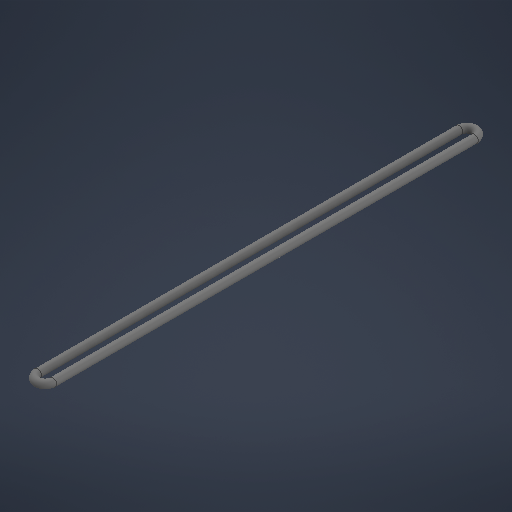
# Autodesk Inventor part: жгут сосало
Saved by Autodesk Inventor 2026.2 (Build 302298000, 298)
## iProperties
Created: 2026-01-20
Part Number: жгут сосало
Material: Типовые
Document SubType Name: Modeling
Designer: GameHD
Density: 1 g/cm^3
Appearance: По умолчанию
Author: GameHD
Autodesk Inventor part; units mm, degrees
ref_plane "YZ Plane" through (0, 0, 0) normal (1, 0, 0) x (0, 1, 0)
ref_plane "XZ Plane" through (0, 0, 0) normal (0, 1, 0) x (-1, 0, 0)
ref_plane "XY Plane" through (0, 0, 0) normal (0, 0, 1) x (1, 0, 0)
sketch "Эскиз1" plane through (0, 0, 0) normal (0, 0, 1) x (1, 0, 0)
  circle A0 centre (0, 0) radius 2.5
  dimension "d0" = 5
  constraints: 1 centre point, 1 coincident
  measures "d0" diameter of A0
sketch "Эскиз2" plane through (0, 0, 0) normal (0, 1, 0) x (-1, 0, 0)
  line L0 (0, 0) -> (-10, 0)
  line L1 (-5, 0) -> (-5, -275)
  line L2 (-5, 0) -> (270, 0) construction
  line L3 (-5, 0) -> (-5, -275) construction
  line L4 (-10, 0) -> (-10, -275)
  line L5 (0, -275) -> (0, 0)
  arc A0 (0, 0) -> (-10, 0) centre (-5, 0) ccw
  arc A1 (-10, -275) -> (0, -275) centre (-5, -275) ccw
  point P0 (-5, -137.5)
  dimension "d1" = 10
  dimension "d2" = 275
  dimension "d3" = 90
  constraints: 14 end point, 4 point on circle, 4 tangent, 3 midpoint, 2 centre point, 2 equal length, 2 horizontal, 1 perpendicular, 1 vertical
  measures "d1" distance of L0.start L0.end
  measures "d2" distance of L1.start L1.end
  measures "d3" angle of L1 L2
sweep "Сдвиг1" add profiles "Эскиз1" path "Эскиз2" path curves L5 A1 L4 A0
